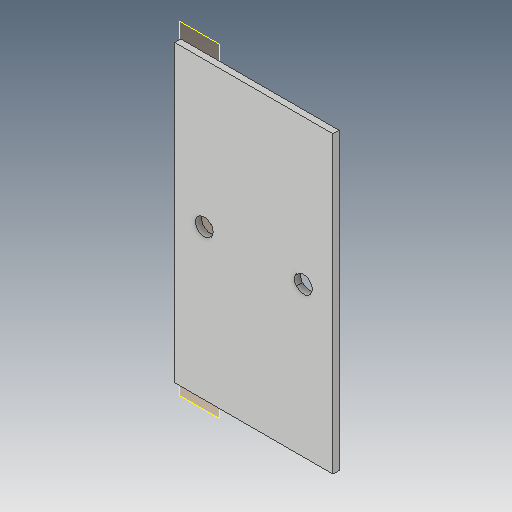
# Autodesk Inventor part: cellSTORM_v5_laser_532nm_adapter
Saved by Autodesk Inventor 2019.4 (Build 234330000, 330)
## iProperties
Created: 2020-05-12
Part Number: cellSTORM_v5_laser_532nm_adapter
Material: Generic
Document SubType Name: Modeling
Designer: diederichbenedict
Density: 1 g/cm^3
Appearance: Default
Author: diederichbenedict
Autodesk Inventor part; units mm, degrees
ref_plane "YZ Plane" through (0, 0, 0) normal (1, 0, 0) x (0, 1, 0)
ref_plane "XZ Plane" through (0, 0, 0) normal (0, 1, 0) x (-1, 0, 0)
ref_plane "XY Plane" through (0, 0, 0) normal (0, 0, 1) x (1, 0, 0)
ref_plane "Work Plane1" through (146.6827, 0.0132, -120.1119) normal (0, 0, 1) x (1, 0, 0)
sketch "Sketch1" plane through (146.6827, 0.0132, -120.1119) normal (0, 0, 1) x (1, 0, 0)
  arc A0 (5.95, 25.2984) -> (5.95, 23.7016) centre (4.8, 24.5) ccw projected
  line L0 (5.95, 25.2984) -> (5.95, 48.23) projected
  line L1 (0, 48.23) -> (5.95, 48.23) projected
  line L2 (0, 0) -> (0, 48.23) projected
  line L3 (5.95, 0) -> (0, 0) projected
  line L4 (5.95, 0) -> (5.95, 23.7016) projected
  arc A1 (19.95, 23.7016) -> (19.95, 25.2984) centre (21.1, 24.5) ccw projected
  line L5 (19.95, 23.7016) -> (19.95, 0) projected
  line L6 (25.9, 0) -> (19.95, 0) projected
  line L7 (25.9, 0) -> (25.9, 48.23) projected
  line L8 (19.95, 48.23) -> (25.9, 48.23) projected
  line L9 (19.95, 48.23) -> (19.95, 25.2984) projected
  line L10 (0, 48.23) -> (25.9, 48.23)
  line L11 (25.9, 48.23) -> (25.9, 0)
  line L12 (25.9, 0) -> (0, 0)
  line L13 (0, 0) -> (0, 48.23)
  circle A2 centre (4.8, 24.5) radius 1.5
  circle A3 centre (21.1, 24.5) radius 1.5
  point P0 (-146.6827, -0.0132)
  dimension "d0" = 3
  dimension "d1" = 3
  constraints: 8 end point, 2 centre point, 2 coincident, 2 parallel, 1 horizontal, 1 perpendicular
  measures "d0" diameter of A2
  measures "d1" diameter of A3
extrude "Extrusion1" add sketch "Sketch1" along normal blind 1 contours A0 L4 A2 L0 | A2 L4 L3 L2 L1 L0 | L0 L10 L9 A3 L5 L12 L4 A2 | L8 L7 L6 L5 A3 L9 | A3 L5 A1 L9 picked at (3.3735, 24.5) picked at (22.5265, 24.5)
body "Solid1"
